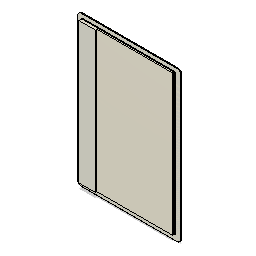
DLT-10inch-Assembly v29 (Autodesk Fusion 360 archive; units mm, degrees)
design "DLT-10Inch-Display+Touchscreen"
Autodesk Fusion 360 part; units mm, degrees
sketch "Sketch1" plane through (0, 0, 0) normal (0, 0, 1) x (1, 0, 0)
  line L0 (78.5, 122.54) -> (-78.5, 122.54)
  line L1 (-84.18, 116.86) -> (-84.18, -116.86)
  line L2 (-78.5, -122.54) -> (78.5, -122.54)
  line L3 (84.18, -116.86) -> (84.18, 116.86)
  line L4 (84.18, 122.54) -> (-84.18, -122.54) construction
  line L5 (-84.18, 122.54) -> (84.18, -122.54) construction
  arc A0 (-84.18, -116.86) -> (-78.5, -122.54) centre (-78.5, -116.86) ccw
  arc A1 (78.5, -122.54) -> (84.18, -116.86) centre (78.5, -116.86) ccw
  arc A2 (84.18, 116.86) -> (78.5, 122.54) centre (78.5, 116.86) ccw
  arc A3 (-78.5, 122.54) -> (-84.18, 116.86) centre (-78.5, 116.86) ccw
  line L6 (-68.18, 108.79) -> (68.18, 108.79)
  line L7 (68.18, 108.79) -> (68.18, -108.79)
  line L8 (68.18, -108.79) -> (-68.18, -108.79)
  line L9 (-68.18, -108.79) -> (-68.18, 108.79)
  dimension "d1" = 168.36
  dimension "d2" = 245.08
  dimension "d3" = 5.68
  dimension "d4" = 5.68
  dimension "d5" = 5.68
  dimension "d6" = 5.68
  dimension "d7" = 136.36
  dimension "d8" = 217.58
  dimension "d9" = 16
  dimension "d10" = 16
  dimension "d11" = 13.75
  dimension "d12" = 13.75
  constraint perpendicular L0 L1
  constraint parallel L0 L2
  constraint parallel L1 L3
  constraint horizontal L0
  constraint coincident L4 origin
  constraint coincident L5 origin
  constraint coincident L4.end L1
  constraint coincident L4.end L2
  constraint tangent L1 A0
  constraint tangent L2 A0
  constraint coincident L5.end L2
  constraint coincident L5.end L3
  constraint tangent L2 A1
  constraint tangent L3 A1
  constraint coincident L4.start L3
  constraint coincident L4.start L0
  constraint tangent L3 A2
  constraint tangent L0 A2
  constraint coincident L5.start L1
  constraint coincident L5.start L0
  constraint tangent L1 A3
  constraint tangent L0 A3
  constraint horizontal L6
  constraint vertical L7
  constraint horizontal L8
  constraint vertical L9
  measures "d1" distance of L4.end L5.end
  measures "d2" distance of L5.start L4.end
  measures "d3" radius of A0
  measures "d4" radius of A1
  measures "d5" radius of A2
  measures "d6" radius of A3
  measures "d7" distance of L6.start L6.end
  measures "d8" distance of L6.start L8.end
  measures "d9" distance of L1 L9
  measures "d10" distance of L3 L7
  measures "d11" distance of L2 L8
  measures "d12" distance of L0 L6
sketch "Sketch2" plane through (0, 0, 0) normal (0, 0, 1) x (1, 0, 0)
  line L0 (67.9, 108.555) -> (-67.9, 108.555)
  line L1 (-67.9, 108.555) -> (-67.9, -108.555)
  line L2 (-67.9, -108.555) -> (67.9, -108.555)
  line L3 (67.9, -108.555) -> (67.9, 108.555)
  line L4 (67.9, 108.555) -> (-67.9, -108.555) construction
  line L5 (-67.9, 108.555) -> (67.9, -108.555) construction
  line L6 (73.8, -114.455) -> (-76.8, -114.455)
  line L7 (-76.8, -114.455) -> (-76.8, 115.555)
  line L8 (-76.8, 115.555) -> (73.8, 115.555)
  line L9 (73.8, 115.555) -> (73.8, -114.455)
  dimension "d13" = 135.8
  dimension "d14" = 217.11
  dimension "d15" = 8.9
  dimension "d16" = 5.9
  dimension "d17" = 7
  dimension "d18" = 5.9
  constraint perpendicular L0 L1
  constraint parallel L0 L2
  constraint parallel L1 L3
  constraint horizontal L0
  constraint coincident L4 origin
  constraint coincident L5 origin
  constraint horizontal L6
  constraint vertical L7
  constraint horizontal L8
  constraint vertical L9
  measures "d13" distance of L1.end L2.end
  measures "d14" distance of L0.end L1.end
  measures "d15" distance of L1 L7
  measures "d16" distance of L3 L9
  measures "d17" distance of L0 L8
  measures "d18" distance of L2 L6
extrude "Extrude1" add sketch "Sketch2" along normal blind 2.25 contours L0 L1 L2 L3 | L6 L7 L8 L9 makes body 1
sketch "Sketch3" plane through (0, 0, 2.25) normal (0, 0, 1) x (1, 0, 0)
  line L0 (73.8, 115.555) -> (-76.8, 115.555)
  line L1 (-76.8, 115.555) -> (-76.8, -114.455)
  line L2 (-76.8, -114.455) -> (73.8, -114.455)
  line L3 (73.8, -114.455) -> (73.8, 115.555)
  line L4 (-76.8, -114.455) -> (-49.8, -114.455)
  line L5 (-49.8, -114.455) -> (-49.8, 115.555)
  line L6 (-49.8, 115.555) -> (-76.8, 115.555)
  line L7 (-76.8, 115.555) -> (-76.8, -114.455)
  dimension "d21" = 27
  constraint horizontal L4
  constraint vertical L5
  constraint horizontal L6
  constraint vertical L7
  constraint coincident L0 L5.end
  constraint coincident L1.end L2.start
  measures "d21" distance of L1.end L4.end
extrude "Extrude2" add sketch "Sketch3" along normal blind 2.35 contours L0 L1 L2 L4 L5 L6 L7 bodies 1
extrude "Extrude3" add sketch "Sketch1" against normal blind 1.55 separate body contours L0 L1 L2 L3 A0 A1 A2 A3 | L6 L7 L8 L9 makes body 2
sketch "Sketch4" plane through (0, 0, 0) normal (0, 0, 1) x (1, 0, 0)
  line L0 (85, 125) -> (75, 125)
  line L1 (75, 125) -> (75, -125)
  line L2 (75, -125) -> (85, -125)
  line L3 (85, -125) -> (85, 125)
  line L4 (85, -125) -> (-100, -125)
  line L5 (-100, -125) -> (-100, -115)
  line L6 (-100, -115) -> (85, -115)
  line L7 (85, -115) -> (85, -125)
  line L8 (-85, -125) -> (-77, -125)
  line L9 (-77, -125) -> (-77, 130)
  line L10 (-77, 130) -> (-85, 130)
  line L11 (-85, 130) -> (-85, -125)
  line L12 (-85, 130) -> (85, 130)
  line L13 (85, 130) -> (85, 116.2681)
  line L14 (85, 116.2681) -> (-85, 116.2681)
  line L15 (-85, 116.2681) -> (-85, 130)
  line L16 (-78.5, -122.54) -> (78.5, -122.54)
  arc A0 (78.5, -122.54) -> (84.18, -116.86) centre (78.5, -116.86) ccw
  line L17 (84.18, -116.86) -> (84.18, 116.86)
  arc A1 (84.18, 116.86) -> (78.5, 122.54) centre (78.5, 116.86) ccw
  line L18 (78.5, 122.54) -> (-78.5, 122.54)
  arc A2 (-78.5, 122.54) -> (-84.18, 116.86) centre (-78.5, 116.86) ccw
  line L19 (-84.18, 116.86) -> (-84.18, -116.86)
  arc A3 (-84.18, -116.86) -> (-78.5, -122.54) centre (-78.5, -116.86) ccw
  dimension "d26" = 5.68
  dimension "d27" = 5.68
  dimension "d28" = 5.68
  dimension "d29" = 5.68
  constraint horizontal L0
  constraint vertical L1
  constraint horizontal L2
  constraint vertical L3
  constraint horizontal L4
  constraint vertical L5
  constraint horizontal L6
  constraint vertical L7
  constraint horizontal L8
  constraint vertical L9
  constraint horizontal L10
  constraint vertical L11
  constraint coincident L4 L8.start
  constraint horizontal L12
  constraint vertical L13
  constraint horizontal L14
  constraint vertical L15
  constraint coincident L3 L13.end
  constraint perpendicular L18 L19
  constraint parallel L16 L18
  constraint parallel L17 L19
  constraint horizontal L18
  constraint tangent L19 A3
  constraint tangent L16 A3
  constraint tangent L16 A0
  constraint tangent A0 L17
  constraint tangent L17 A1
  constraint tangent A1 L18
  constraint tangent A2 L19
  constraint tangent L18 A2
  measures "d26" radius of A3
  measures "d27" radius of A0
  measures "d28" radius of A1
  measures "d29" radius of A2
extrude "Extrude4" add sketch "Sketch4" along normal blind 0.25 separate body contours L1 L14 L17 A1 L18 | L1 L9 L14 L18 | L1 L6 L14 L17 | L9 L14 L18 A2 L19 | L1 L6 L16 A0 L17 | L1 L6 L9 L16 | L6 L9 L14 L19 | L6 L9 L16 L19 A3 makes body 3
move_body "Move1" bodies 1 to x (1, 0, 0) y (0, 1, 0) z (0, 0, 1) at (0, 0, 0.8)
equation "d13 = 135.5 mm + 0.3 mm"
equation "d14 = 216.81 mm + 0.3 mm"
equation "d22 = 4.6 mm - 2.25 mm"
named bodies: "LCD", "Touchscreen", "Adhesive"
